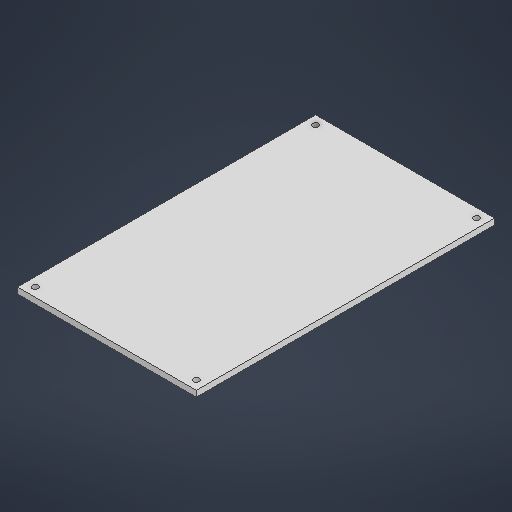
# Autodesk Inventor part: Part3
Saved by Autodesk Inventor 2026.2 (Build 302298000, 298)
## iProperties
Created: 2026-04-03
Part Number: Part3
Material: Generic
Document SubType Name: Modeling
Designer: Octa
Density: 1 g/cm^3
Appearance: Default
Author: Octa
Autodesk Inventor part; units mm, degrees
ref_plane "YZ Plane" through (0, 0, 0) normal (1, 0, 0) x (0, 1, 0)
ref_plane "XZ Plane" through (0, 0, 0) normal (0, 1, 0) x (-1, 0, 0)
ref_plane "XY Plane" through (0, 0, 0) normal (0, 0, 1) x (1, 0, 0)
sketch "Sketch1" plane through (0, 0, 0) normal (0, 1, 0) x (-1, 0, 0)
  line L0 (0, 0) -> (-60, 0)
  line L1 (-60, 0) -> (-60, -100)
  line L2 (-60, -100) -> (0, -100)
  line L3 (0, -100) -> (0, 0)
  line L4 (-58, -5) -> (-58, -95)
  line L5 (-5, -2) -> (-5, -3)
  line L6 (-3, -5) -> (-2, -5)
  line L7 (-55, -2) -> (-55, -3)
  line L8 (-57, -5) -> (-58, -5)
  line L9 (-55, -98) -> (-55, -97)
  line L10 (-57, -95) -> (-58, -95)
  line L11 (-5, -98) -> (-5, -97)
  line L12 (-3, -95) -> (-2, -95)
  arc A0 (-5, -3) -> (-3, -5) centre (-3, -3) ccw
  arc A1 (-57, -5) -> (-55, -3) centre (-57, -3) ccw
  arc A2 (-55, -97) -> (-57, -95) centre (-57, -97) ccw
  arc A3 (-3, -95) -> (-5, -97) centre (-3, -97) ccw
  circle A4 centre (-57, -3) radius 1
  circle A5 centre (-57, -97) radius 1
  circle A6 centre (-3, -97) radius 1
  circle A7 centre (-3, -3) radius 1
  line L13 (-5, -2) -> (-55, -2)
  line L14 (-2, -95) -> (-2, -5)
  line L15 (-55, -98) -> (-5, -98)
  point P0 (-5, -5)
  point P1 (-55, -5)
  point P2 (-55, -95)
  point P3 (-5, -95)
  dimension "d0" = 60
  dimension "d1" = 100
  dimension "d6" = 3
  dimension "d7" = 3
  dimension "d8" = 3
  dimension "d9" = 3
  dimension "d10" = 3
  dimension "d11" = 3
  dimension "d12" = 2
  dimension "d13" = 3
  dimension "d14" = 2
  dimension "d15" = 2
  dimension "d16" = 2
  dimension "d17" = 2
  constraints: 32 end point, 9 point on line, 8 centre point, 8 point on circle, 8 tangent, 4 coincident, 4 parallel, 2 equal radius, 2 horizontal, 2 perpendicular
  measures "d0" distance of L2.end L1.end
  measures "d1" distance of L1.end L0.end
  measures "d6" distance of L6.end point (-5, -5)
  measures "d7" distance of point (-5, -5) L5.start
  measures "d8" distance of L4.start point (-55, -5)
  measures "d9" distance of L4.end point (-55, -95)
  measures "d10" distance of point (-5, -95) L12.end
  measures "d11" distance of L11.start point (-5, -95)
  measures "d12" radius of A0
  measures "d13" distance of L9.start point (-55, -95)
  measures "d14" radius of A2
  measures "d15" diameter of A4
  measures "d16" diameter of A6
  measures "d17" diameter of A7
extrude "Extrusion1" add sketch "Sketch1" along normal blind 2 contours L3 L2 L1 L0 | L8 A1 L7 L13 L5 A0 L6 L14 L12 A3 L11 L15 L9 A2 L10 L4
body "Solid1"
